Autodesk Fusion 360 part; units mm, degrees
(part 2 of 8)
  spline S26 degree 5 poles (-199.3182, -646.9433) (-199.2305, -646.913) (-199.0552, -646.8523) (-198.7925, -646.7608) (-198.4427, -646.6379) (-198.0064, -646.4828) (-197.571, -646.3262) (-197.1366, -646.1681) (-196.703, -646.0086) (-196.2703, -645.8476) (-195.8386, -645.6851) (-195.4078, -645.521) (-194.9779, -645.3555) (-194.549, -645.1885) (-194.1211, -645.0199) (-193.6942, -644.8498) (-193.2682, -644.6782) (-192.8433, -644.505) (-192.4194, -644.3303) (-191.9965, -644.154) (-191.5747, -643.9761) (-191.1539, -643.7966) (-190.7342, -643.6156) (-190.3155, -643.4329) (-189.898, -643.2486) (-189.4816, -643.0627) (-189.0663, -642.8752) (-188.6521, -642.686) (-188.2391, -642.4951) (-187.8273, -642.3026) (-187.4167, -642.1083) (-187.0073, -641.9124) (-186.599, -641.7148) (-186.1921, -641.5154) (-185.7864, -641.3143) (-185.382, -641.1114) (-184.9788, -640.9068) (-184.577, -640.7003) (-184.1766, -640.492) (-183.7775, -640.2819) (-183.3798, -640.07) (-182.9836, -639.8562) (-182.5887, -639.6404) (-182.1954, -639.4228) (-181.8035, -639.2033) (-181.4131, -638.9817) (-181.0244, -638.7582) (-180.6372, -638.5326) (-180.2517, -638.3049) (-179.8679, -638.0751) (-179.4858, -637.8433) (-179.1054, -637.6093) (-178.7267, -637.3731) (-178.3499, -637.1347) (-177.975, -636.8941) (-177.602, -636.651) (-177.2312, -636.4055) (-176.8625, -636.1574) (-176.4961, -635.9068) (-176.1319, -635.6535) (-175.77, -635.3976) (-175.4104, -635.1391) (-175.053, -634.8779) (-174.7334, -634.64) (-174.4864, -634.4531) (-174.3108, -634.3184) (-174.2058, -634.237) (-174.1705, -634.2097) knots -1 -1 -1 -1 -1 -1 -0.98571429 -0.97142857 -0.95714286 -0.94285714 -0.92857143 -0.91428571 -0.9 -0.88571429 -0.87142857 -0.85714286 -0.84285714 -0.82857143 -0.81428571 -0.8 -0.78571429 -0.77142857 -0.75714286 -0.74285714 -0.72857143 -0.71428571 -0.7 -0.68571429 -0.67142857 -0.65714286 -0.64285714 -0.62857143 -0.61428571 -0.6 -0.58571429 -0.57142857 -0.55714286 -0.54285714 -0.52857143 -0.51428571 -0.5 -0.48571429 -0.47142857 -0.45714286 -0.44285714 -0.42857143 -0.41428571 -0.4 -0.38571429 -0.37142857 -0.35714286 -0.34285714 -0.32857143 -0.31428571 -0.3 -0.28571429 -0.27142857 -0.25714286 -0.24285714 -0.22857143 -0.21428571 -0.2 -0.18571429 -0.17142857 -0.15714286 -0.14285714 -0.12857143 -0.11428571 -0.10707295 -0.10707295 -0.10707295 -0.10707295 -0.10707295 -0.10707295
  spline S27 degree 3 poles (-172.1165, -634.3004) (-172.268, -634.1598) (-172.4455, -634.05) (-172.8326, -633.9047) (-173.0384, -633.8705) (-173.412, -633.8819) (-173.5771, -633.9132) (-173.8914, -634.0263) (-174.0386, -634.1073) (-174.1705, -634.2097) knots 0 0 0 0 0.062015 0.062015 0.12403 0.12403 0.174133 0.174133 0.224236 0.224236 0.224236 0.224236
  arc A14 (-172.1165, -634.3004) -> (-165.887, -639.9095) centre (11.949, -436.1388) ccw
  spline S28 degree 3 poles (-165.5821, -641.9428) (-165.4731, -641.7671) (-165.3994, -641.5719) (-165.331, -641.1642) (-165.337, -640.9556) (-165.4198, -640.5911) (-165.4822, -640.4351) (-165.6535, -640.1483) (-165.7612, -640.0193) (-165.887, -639.9095) knots 0 0 0 0 0.062015 0.062015 0.12403 0.12403 0.174133 0.174133 0.224236 0.224236 0.224236 0.224236
  spline S29 degree 5 poles (-165.5821, -641.9428) (-165.6056, -641.9807) (-165.6755, -642.0937) (-165.7911, -642.2823) (-165.9512, -642.5475) (-166.1544, -642.8903) (-166.3768, -643.273) (-166.5963, -643.6576) (-166.8129, -644.0443) (-167.0268, -644.433) (-167.2378, -644.8236) (-167.4459, -645.2162) (-167.6513, -645.6106) (-167.8541, -646.0069) (-168.0542, -646.405) (-168.2519, -646.8047) (-168.4472, -647.2059) (-168.6402, -647.6087) (-168.8308, -648.013) (-169.0192, -648.4187) (-169.2053, -648.8259) (-169.3892, -649.2345) (-169.5709, -649.6445) (-169.7504, -650.0559) (-169.9278, -650.4685) (-170.1031, -650.8825) (-170.2764, -651.2977) (-170.4476, -651.7142) (-170.6169, -652.1319) (-170.7841, -652.5507) (-170.9494, -652.9707) (-171.1127, -653.3919) (-171.2741, -653.8142) (-171.4336, -654.2376) (-171.5912, -654.6621) (-171.7469, -655.0877) (-171.9008, -655.5143) (-172.0529, -655.942) (-172.2031, -656.3707) (-172.3515, -656.8004) (-172.4982, -657.2311) (-172.6431, -657.6627) (-172.7862, -658.0953) (-172.9275, -658.5289) (-173.0672, -658.9634) (-173.2051, -659.3989) (-173.3413, -659.8352) (-173.4758, -660.2724) (-173.6086, -660.7106) (-173.7397, -661.1495) (-173.8692, -661.5894) (-173.997, -662.0301) (-174.1232, -662.4716) (-174.2477, -662.914) (-174.3706, -663.3572) (-174.4919, -663.8012) (-174.6116, -664.246) (-174.7297, -664.6916) (-174.8462, -665.138) (-174.9611, -665.5851) (-175.0744, -666.033) (-175.1862, -666.4816) (-175.2964, -666.931) (-175.405, -667.3811) (-175.4907, -667.7418) (-175.5543, -668.0126) (-175.5964, -668.1933) (-175.6173, -668.2837) knots 0.10707295 0.10707295 0.10707295 0.10707295 0.10707295 0.10707295 0.11428571 0.12857143 0.14285714 0.15714286 0.17142857 0.18571429 0.2 0.21428571 0.22857143 0.24285714 0.25714286 0.27142857 0.28571429 0.3 0.31428571 0.32857143 0.34285714 0.35714286 0.37142857 0.38571429 0.4 0.41428571 0.42857143 0.44285714 0.45714286 0.47142857 0.48571429 0.5 0.51428571 0.52857143 0.54285714 0.55714286 0.57142857 0.58571429 0.6 0.61428571 0.62857143 0.64285714 0.65714286 0.67142857 0.68571429 0.7 0.71428571 0.72857143 0.74285714 0.75714286 0.77142857 0.78571429 0.8 0.81428571 0.82857143 0.84285714 0.85714286 0.87142857 0.88571429 0.9 0.91428571 0.92857143 0.94285714 0.95714286 0.97142857 0.98571429 1 1 1 1 1 1
  arc A15 (-175.6173, -668.2837) -> (-167.9238, -674.2945) centre (11.949, -436.1388) ccw
  spline S30 degree 5 poles (-167.9238, -674.2945) (-167.8412, -674.2523) (-167.6761, -674.1678) (-167.4286, -674.0406) (-167.0994, -673.8702) (-166.6889, -673.6559) (-166.2796, -673.4402) (-165.8713, -673.2232) (-165.4641, -673.0049) (-165.0581, -672.7852) (-164.6532, -672.5642) (-164.2494, -672.3418) (-163.8468, -672.1181) (-163.4453, -671.893) (-163.045, -671.6665) (-162.6459, -671.4387) (-162.248, -671.2094) (-161.8513, -670.9788) (-161.4558, -670.7468) (-161.0616, -670.5133) (-160.6686, -670.2785) (-160.2769, -670.0422) (-159.8865, -669.8045) (-159.4974, -669.5653) (-159.1095, -669.3247) (-158.723, -669.0827) (-158.3379, -668.8391) (-157.9541, -668.5941) (-157.5717, -668.3477) (-157.1907, -668.0997) (-156.811, -667.8502) (-156.4329, -667.5992) (-156.0561, -667.3467) (-155.6809, -667.0926) (-155.3071, -666.837) (-154.9349, -666.5798) (-154.5641, -666.321) (-154.195, -666.0607) (-153.8274, -665.7987) (-153.4615, -665.5351) (-153.0972, -665.2699) (-152.7345, -665.003) (-152.3735, -664.7344) (-152.0143, -664.4641) (-151.6568, -664.1922) (-151.3011, -663.9185) (-150.9472, -663.643) (-150.5952, -663.3657) (-150.2452, -663.0866) (-149.897, -662.8057) (-149.5509, -662.5229) (-149.2068, -662.2382) (-148.8647, -661.9516) (-148.5247, -661.6631) (-148.1869, -661.3726) (-147.8514, -661.0801) (-147.5183, -660.7853) (-147.1878, -660.4884) (-146.8598, -660.1891) (-146.5344, -659.8876) (-146.2117, -659.5838) (-145.8915, -659.2778) (-145.574, -658.9694) (-145.2905, -658.6894) (-145.072, -658.4699) (-144.9169, -658.3121) (-144.8242, -658.2169) (-144.7931, -658.1849) knots -1 -1 -1 -1 -1 -1 -0.98571429 -0.97142857 -0.95714286 -0.94285714 -0.92857143 -0.91428571 -0.9 -0.88571429 -0.87142857 -0.85714286 -0.84285714 -0.82857143 -0.81428571 -0.8 -0.78571429 -0.77142857 -0.75714286 -0.74285714 -0.72857143 -0.71428571 -0.7 -0.68571429 -0.67142857 -0.65714286 -0.64285714 -0.62857143 -0.61428571 -0.6 -0.58571429 -0.57142857 -0.55714286 -0.54285714 -0.52857143 -0.51428571 -0.5 -0.48571429 -0.47142857 -0.45714286 -0.44285714 -0.42857143 -0.41428571 -0.4 -0.38571429 -0.37142857 -0.35714286 -0.34285714 -0.32857143 -0.31428571 -0.3 -0.28571429 -0.27142857 -0.25714286 -0.24285714 -0.22857143 -0.21428571 -0.2 -0.18571429 -0.17142857 -0.15714286 -0.14285714 -0.12857143 -0.11428571 -0.10707295 -0.10707295 -0.10707295 -0.10707295 -0.10707295 -0.10707295
  spline S31 degree 3 poles (-142.7465, -657.9889) (-142.916, -657.8707) (-143.1071, -657.7867) (-143.5106, -657.6967) (-143.7192, -657.6915) (-144.0875, -657.7547) (-144.2467, -657.8088) (-144.5422, -657.9644) (-144.6767, -658.0651) (-144.7931, -658.1849) knots 0 0 0 0 0.062015 0.062015 0.12403 0.12403 0.174133 0.174133 0.224236 0.224236 0.224236 0.224236
  arc A16 (-142.7465, -657.9889) -> (-135.7969, -662.6764) centre (11.949, -436.1388) ccw
  spline S32 degree 3 poles (-135.212, -664.6475) (-135.1285, -664.4584) (-135.0827, -664.2548) (-135.0717, -663.8415) (-135.1067, -663.6357) (-135.2394, -663.2864) (-135.3229, -663.1406) (-135.5324, -662.8804) (-135.657, -662.7677) (-135.7969, -662.6764) knots 0 0 0 0 0.062015 0.062015 0.12403 0.12403 0.174133 0.174133 0.224236 0.224236 0.224236 0.224236
  spline S33 degree 5 poles (-135.212, -664.6475) (-135.23, -664.6882) (-135.2835, -664.8099) (-135.3717, -665.0128) (-135.4934, -665.2977) (-135.6468, -665.6654) (-135.8138, -666.0753) (-135.9776, -666.4868) (-136.1384, -666.8999) (-136.296, -667.3145) (-136.4506, -667.7306) (-136.6021, -668.1484) (-136.7506, -668.5676) (-136.8962, -668.9883) (-137.039, -669.4103) (-137.1792, -669.8336) (-137.3167, -670.2581) (-137.4518, -670.6839) (-137.5843, -671.1107) (-137.7144, -671.5387) (-137.842, -671.9679) (-137.9672, -672.3981) (-138.0901, -672.8294) (-138.2106, -673.2617) (-138.3289, -673.6951) (-138.4449, -674.1294) (-138.5587, -674.5647) (-138.6703, -675.0009) (-138.7797, -675.4381) (-138.887, -675.8761) (-138.9922, -676.3151) (-139.0954, -676.7549) (-139.1964, -677.1955) (-139.2954, -677.637) (-139.3924, -678.0793) (-139.4874, -678.5224) (-139.5804, -678.9663) (-139.6715, -679.411) (-139.7606, -679.8564) (-139.8478, -680.3026) (-139.9331, -680.7495) (-140.0164, -681.1971) (-140.0979, -681.6454) (-140.1776, -682.0945) (-140.2554, -682.5442) (-140.3314, -682.9946) (-140.4055, -683.4456) (-140.4778, -683.8973) (-140.5484, -684.3497) (-140.6172, -684.8026) (-140.6841, -685.2562) (-140.7494, -685.7104) (-140.8129, -686.1652) (-140.8746, -686.6206) (-140.9347, -687.0766) (-140.993, -687.5332) (-141.0496, -687.9903) (-141.1045, -688.448) (-141.1577, -688.9062) (-141.2093, -689.365) (-141.2592, -689.8243) (-141.3075, -690.2841) (-141.354, -690.7445) (-141.399, -691.2053) (-141.4337, -691.5744) (-141.4589, -691.8515) (-141.4754, -692.0363) (-141.4836, -692.1287) knots 0.10707295 0.10707295 0.10707295 0.10707295 0.10707295 0.10707295 0.11428571 0.12857143 0.14285714 0.15714286 0.17142857 0.18571429 0.2 0.21428571 0.22857143 0.24285714 0.25714286 0.27142857 0.28571429 0.3 0.31428571 0.32857143 0.34285714 0.35714286 0.37142857 0.38571429 0.4 0.41428571 0.42857143 0.44285714 0.45714286 0.47142857 0.48571429 0.5 0.51428571 0.52857143 0.54285714 0.55714286 0.57142857 0.58571429 0.6 0.61428571 0.62857143 0.64285714 0.65714286 0.67142857 0.68571429 0.7 0.71428571 0.72857143 0.74285714 0.75714286 0.77142857 0.78571429 0.8 0.81428571 0.82857143 0.84285714 0.85714286 0.87142857 0.88571429 0.9 0.91428571 0.92857143 0.94285714 0.95714286 0.97142857 0.98571429 1 1 1 1 1 1
  arc A17 (-141.4836, -692.1287) -> (-133.0285, -697.0103) centre (11.949, -436.1388) ccw
  spline S34 degree 5 poles (-133.0285, -697.0103) (-132.9525, -696.957) (-132.8007, -696.8503) (-132.5734, -696.6899) (-132.2711, -696.4753) (-131.8945, -696.2059) (-131.5191, -695.9354) (-131.145, -695.6637) (-130.7722, -695.3909) (-130.4007, -695.1168) (-130.0304, -694.8416) (-129.6615, -694.5652) (-129.2939, -694.2876) (-128.9277, -694.0088) (-128.5628, -693.7289) (-128.1993, -693.4477) (-127.8372, -693.1653) (-127.4765, -692.8817) (-127.1171, -692.5969) (-126.7592, -692.3108) (-126.4028, -692.0236) (-126.0478, -691.7351) (-125.6942, -691.4453) (-125.3422, -691.1543) (-124.9916, -690.8621) (-124.6425, -690.5686) (-124.295, -690.2739) (-123.9491, -689.9778) (-123.6047, -689.6805) (-123.2619, -689.3819) (-122.9207, -689.0821) (-122.5811, -688.7809) (-122.2432, -688.4784) (-121.907, -688.1746) (-121.5724, -687.8694) (-121.2396, -687.5629) (-120.9085, -687.2551) (-120.5791, -686.9459) (-120.2516, -686.6353) (-119.9259, -686.3233) (-119.6021, -686.01) (-119.2801, -685.6952) (-118.96, -685.379) (-118.6418, -685.0614) (-118.3257, -684.7423) (-118.0115, -684.4218) (-117.6994, -684.0997) (-117.3895, -683.7761) (-117.0817, -683.451) (-116.776, -683.1244) (-116.4726, -682.7962) (-116.1715, -682.4664) (-115.8726, -682.135) (-115.576, -681.802) (-115.282, -681.4673) (-114.9905, -681.1309) (-114.7016, -680.7926) (-114.4156, -680.4526) (-114.1325, -680.1106) (-113.8523, -679.7667) (-113.5749, -679.421) (-113.3005, -679.0734) (-113.029, -678.7238) (-112.7872, -678.4071) (-112.6013, -678.1593) (-112.4697, -677.9814) (-112.3912, -677.8742) (-112.3648, -677.8383) knots -1 -1 -1 -1 -1 -1 -0.98571429 -0.97142857 -0.95714286 -0.94285714 -0.92857143 -0.91428571 -0.9 -0.88571429 -0.87142857 -0.85714286 -0.84285714 -0.82857143 -0.81428571 -0.8 -0.78571429 -0.77142857 -0.75714286 -0.74285714 -0.72857143 -0.71428571 -0.7 -0.68571429 -0.67142857 -0.65714286 -0.64285714 -0.62857143 -0.61428571 -0.6 -0.58571429 -0.57142857 -0.55714286 -0.54285714 -0.52857143 -0.51428571 -0.5 -0.48571429 -0.47142857 -0.45714286 -0.44285714 -0.42857143 -0.41428571 -0.4 -0.38571429 -0.37142857 -0.35714286 -0.34285714 -0.32857143 -0.31428571 -0.3 -0.28571429 -0.27142857 -0.25714286 -0.24285714 -0.22857143 -0.21428571 -0.2 -0.18571429 -0.17142857 -0.15714286 -0.14285714 -0.12857143 -0.11428571 -0.10707295 -0.10707295 -0.10707295 -0.10707295 -0.10707295 -0.10707295
  spline S35 degree 3 poles (-110.3654, -677.3593) (-110.5498, -677.2658) (-110.7506, -677.2093) (-111.1627, -677.1763) (-111.3701, -677.2002) (-111.726, -677.314) (-111.8761, -677.3897) (-112.147, -677.585) (-112.2663, -677.7034) (-112.3648, -677.8383) knots 0 0 0 0 0.062015 0.062015 0.12403 0.12403 0.174133 0.174133 0.224236 0.224236 0.224236 0.224236
  arc A18 (-110.3654, -677.3593) -> (-102.8311, -681.034) centre (11.949, -436.1388) ccw
  spline S36 degree 3 poles (-101.9775, -682.9045) (-101.9212, -682.7056) (-101.9042, -682.4976) (-101.9508, -682.0868) (-102.0141, -681.888) (-102.1941, -681.5604) (-102.2972, -681.4277) (-102.5408, -681.1992) (-102.6799, -681.1049) (-102.8311, -681.034) knots 0 0 0 0 0.062015 0.062015 0.12403 0.12403 0.174133 0.174133 0.224236 0.224236 0.224236 0.224236
  spline S37 degree 5 poles (-101.9775, -682.9045) (-101.9897, -682.9474) (-102.0258, -683.0753) (-102.0849, -683.2885) (-102.1657, -683.5875) (-102.2665, -683.973) (-102.3748, -684.4022) (-102.4798, -684.8325) (-102.5815, -685.2639) (-102.6799, -685.6964) (-102.7751, -686.1301) (-102.8669, -686.5648) (-102.9557, -687.0006) (-103.0413, -687.4375) (-103.124, -687.8752) (-103.2038, -688.3139) (-103.281, -688.7535) (-103.3554, -689.1938) (-103.4273, -689.635) (-103.4965, -690.077) (-103.5632, -690.5197) (-103.6273, -690.9631) (-103.689, -691.4073) (-103.7482, -691.8522) (-103.8049, -692.2978) (-103.8594, -692.7441) (-103.9115, -693.191) (-103.9613, -693.6385) (-104.0088, -694.0866) (-104.0541, -694.5353) (-104.0972, -694.9846) (-104.1381, -695.4345) (-104.1769, -695.885) (-104.2135, -696.3359) (-104.248, -696.7874) (-104.2803, -697.2394) (-104.3107, -697.692) (-104.339, -698.145) (-104.3652, -698.5985) (-104.3895, -699.0524) (-104.4117, -699.5069) (-104.432, -699.9617) (-104.4503, -700.417) (-104.4667, -700.8728) (-104.4811, -701.3289) (-104.4937, -701.7855) (-104.5043, -702.2425) (-104.5131, -702.6999) (-104.52, -703.1576) (-104.5251, -703.6158) (-104.5283, -704.0743) (-104.5297, -704.5331) (-104.5293, -704.9923) (-104.527, -705.4519) (-104.523, -705.9118) (-104.5172, -706.372) (-104.5097, -706.8326) (-104.5003, -707.2935) (-104.4893, -707.7546) (-104.4765, -708.2161) (-104.462, -708.6779) (-104.4458, -709.14) (-104.4278, -709.6023) (-104.4082, -710.0649) (-104.3912, -710.4353) (-104.3776, -710.7131) (-104.3683, -710.8984) (-104.3635, -710.9911) knots 0.10707295 0.10707295 0.10707295 0.10707295 0.10707295 0.10707295 0.11428571 0.12857143 0.14285714 0.15714286 0.17142857 0.18571429 0.2 0.21428571 0.22857143 0.24285714 0.25714286 0.27142857 0.28571429 0.3 0.31428571 0.32857143 0.34285714 0.35714286 0.37142857 0.38571429 0.4 0.41428571 0.42857143 0.44285714 0.45714286 0.47142857 0.48571429 0.5 0.51428571 0.52857143 0.54285714 0.55714286 0.57142857 0.58571429 0.6 0.61428571 0.62857143 0.64285714 0.65714286 0.67142857 0.68571429 0.7 0.71428571 0.72857143 0.74285714 0.75714286 0.77142857 0.78571429 0.8 0.81428571 0.82857143 0.84285714 0.85714286 0.87142857 0.88571429 0.9 0.91428571 0.92857143 0.94285714 0.95714286 0.97142857 0.98571429 1 1 1 1 1 1
  arc A19 (-104.3635, -710.9911) -> (-95.3113, -714.6484) centre (11.949, -436.1388) ccw
  spline S38 degree 5 poles (-95.3113, -714.6484) (-95.2435, -714.5851) (-95.108, -714.4583) (-94.9052, -714.2678) (-94.6357, -714.0133) (-94.3002, -713.6941) (-93.9662, -713.374) (-93.6335, -713.0529) (-93.3023, -712.7308) (-92.9725, -712.4077) (-92.6442, -712.0836) (-92.3174, -711.7586) (-91.992, -711.4325) (-91.6681, -711.1055) (-91.3458, -710.7775) (-91.0249, -710.4484) (-90.7056, -710.1184) (-90.3879, -709.7874) (-90.0717, -709.4553) (-89.7571, -709.1222) (-89.4441, -708.7882) (-89.1327, -708.4531) (-88.8229, -708.1169) (-88.5147, -707.7798) (-88.2083, -707.4416) (-87.9034, -707.1024) (-87.6003, -706.7622) (-87.2989, -706.4209) (-86.9993, -706.0785) (-86.7014, -705.7351) (-86.4052, -705.3907) (-86.1109, -705.0452) (-85.8184, -704.6986) (-85.5277, -704.3509) (-85.2388, -704.0022) (-84.9519, -703.6523) (-84.6669, -703.3014) (-84.3838, -702.9494) (-84.1027, -702.5962) (-83.8236, -702.242) (-83.5465, -701.8866) (-83.2714, -701.5301) (-82.9985, -701.1724) (-82.7276, -700.8136) (-82.4589, -700.4536) (-82.1924, -700.0925) (-81.9282, -699.7301) (-81.6663, -699.3666) (-81.4067, -699.0018) (-81.1495, -698.6358) (-80.8948, -698.2685) (-80.6424, -697.9001) (-80.3926, -697.5303) (-80.1453, -697.1592) (-79.9006, -696.7869) (-79.6588, -696.4132) (-79.4198, -696.038) (-79.184, -695.6615) (-78.9512, -695.2834) (-78.7215, -694.9039) (-78.495, -694.523) (-78.2716, -694.1405) (-78.0514, -693.7566) (-77.8561, -693.4093) (-77.7065, -693.138) (-77.6009, -692.9435) (-77.538, -692.8265) (-77.517, -692.7872) knots -1 -1 -1 -1 -1 -1 -0.98571429 -0.97142857 -0.95714286 -0.94285714 -0.92857143 -0.91428571 -0.9 -0.88571429 -0.87142857 -0.85714286 -0.84285714 -0.82857143 -0.81428571 -0.8 -0.78571429 -0.77142857 -0.75714286 -0.74285714 -0.72857143 -0.71428571 -0.7 -0.68571429 -0.67142857 -0.65714286 -0.64285714 -0.62857143 -0.61428571 -0.6 -0.58571429 -0.57142857 -0.55714286 -0.54285714 -0.52857143 -0.51428571 -0.5 -0.48571429 -0.47142857 -0.45714286 -0.44285714 -0.42857143 -0.41428571 -0.4 -0.38571429 -0.37142857 -0.35714286 -0.34285714 -0.32857143 -0.31428571 -0.3 -0.28571429 -0.27142857 -0.25714286 -0.24285714 -0.22857143 -0.21428571 -0.2 -0.18571429 -0.17142857 -0.15714286 -0.14285714 -0.12857143 -0.11428571 -0.10707295 -0.10707295 -0.10707295 -0.10707295 -0.10707295 -0.10707295
  spline S39 degree 3 poles (-75.6036, -692.0347) (-75.7992, -691.9678) (-76.006, -691.9397) (-76.4187, -691.9644) (-76.6207, -692.0169) (-76.9573, -692.1792) (-77.0954, -692.275) (-77.3365, -692.5061) (-77.4381, -692.64) (-77.517, -692.7872) knots 0 0 0 0 0.062015 0.062015 0.12403 0.12403 0.174133 0.174133 0.224236 0.224236 0.224236 0.224236
  arc A20 (-75.6036, -692.0347) -> (-67.6313, -694.625) centre (11.949, -436.1388) ccw
  spline S40 degree 3 poles (-66.5257, -696.3585) (-66.4975, -696.1537) (-66.5096, -695.9454) (-66.613, -695.5451) (-66.7033, -695.3569) (-66.9272, -695.0577) (-67.0477, -694.9406) (-67.3208, -694.7482) (-67.4716, -694.6742) (-67.6313, -694.625) knots 0 0 0 0 0.062015 0.062015 0.12403 0.12403 0.174133 0.174133 0.224236 0.224236 0.224236 0.224236
  spline S41 degree 5 poles (-66.5257, -696.3585) (-66.5317, -696.4026) (-66.5496, -696.5343) (-66.5785, -696.7537) (-66.617, -697.0611) (-66.6631, -697.4569) (-66.7106, -697.8969) (-66.7547, -698.3376) (-66.7953, -698.779) (-66.8326, -699.221) (-66.8665, -699.6637) (-66.897, -700.107) (-66.9242, -700.5509) (-66.9482, -700.9954) (-66.9692, -701.4404) (-66.9872, -701.886) (-67.0024, -702.332) (-67.0148, -702.7784) (-67.0246, -703.2253) (-67.0316, -703.6726) (-67.0361, -704.1202) (-67.0379, -704.5683) (-67.0371, -705.0168) (-67.0338, -705.4656) (-67.028, -705.9147) (-67.0198, -706.3642) (-67.0092, -706.814) (-66.9962, -707.2641) (-66.9809, -707.7145) (-66.9633, -708.1652) (-66.9435, -708.6161) (-66.9214, -709.0673) (-66.897, -709.5187) (-66.8705, -709.9704) (-66.8418, -710.4223) (-66.811, -710.8744) (-66.7781, -711.3268) (-66.743, -711.7793) (-66.7059, -712.232) (-66.6668, -712.685) (-66.6255, -713.1381) (-66.5823, -713.5913) (-66.5371, -714.0448) (-66.4899, -714.4983) (-66.4407, -714.9521) (-66.3896, -715.406) (-66.3365, -715.86) (-66.2816, -716.3141) (-66.2247, -716.7684) (-66.1659, -717.2227) (-66.1053, -717.6772) (-66.0428, -718.1318) (-65.9785, -718.5865) (-65.9123, -719.0413) (-65.8444, -719.4962) (-65.7746, -719.9511) (-65.703, -720.4061) (-65.6296, -720.8612) (-65.5545, -721.3164) (-65.4776, -721.7716) (-65.399, -722.2268) (-65.3186, -722.6822) (-65.2365, -723.1375) (-65.1527, -723.5929) (-65.0843, -723.9573) (-65.0322, -724.2305) (-64.9971, -724.4127) (-64.9795, -724.5038) knots 0.10707295 0.10707295 0.10707295 0.10707295 0.10707295 0.10707295 0.11428571 0.12857143 0.14285714 0.15714286 0.17142857 0.18571429 0.2 0.21428571 0.22857143 0.24285714 0.25714286 0.27142857 0.28571429 0.3 0.31428571 0.32857143 0.34285714 0.35714286 0.37142857 0.38571429 0.4 0.41428571 0.42857143 0.44285714 0.45714286 0.47142857 0.48571429 0.5 0.51428571 0.52857143 0.54285714 0.55714286 0.57142857 0.58571429 0.6 0.61428571 0.62857143 0.64285714 0.65714286 0.67142857 0.68571429 0.7 0.71428571 0.72857143 0.74285714 0.75714286 0.77142857 0.78571429 0.8 0.81428571 0.82857143 0.84285714 0.85714286 0.87142857 0.88571429 0.9 0.91428571 0.92857143 0.94285714 0.95714286 0.97142857 0.98571429 1 1 1 1 1 1
  arc A21 (-64.9795, -724.5038) -> (-55.5064, -726.8657) centre (11.949, -436.1388) ccw
  spline S42 degree 5 poles (-55.5064, -726.8657) (-55.448, -726.7936) (-55.3315, -726.6492) (-55.1572, -726.4323) (-54.9258, -726.1428) (-54.638, -725.78) (-54.3517, -725.4165) (-54.067, -725.0522) (-53.7838, -724.6872) (-53.5022, -724.3213) (-53.2222, -723.9547) (-52.9438, -723.5874) (-52.667, -723.2192) (-52.3918, -722.8503) (-52.1182, -722.4806) (-51.8463, -722.1101) (-51.576, -721.7388) (-51.3074, -721.3668) (-51.0405, -720.9939) (-50.7753, -720.6203) (-50.5119, -720.2459) (-50.2501, -719.8708) (-49.9901, -719.4948) (-49.7319, -719.118) (-49.4755, -718.7405) (-49.2208, -718.3622) (-48.968, -717.9831) (-48.7171, -717.6031) (-48.468, -717.2224) (-48.2208, -716.8409) (-47.9754, -716.4586) (-47.732, -716.0755) (-47.4906, -715.6915) (-47.2511, -715.3068) (-47.0136, -714.9213) (-46.7782, -714.5349) (-46.5448, -714.1477) (-46.3134, -713.7597) (-46.0842, -713.3709) (-45.8571, -712.9813) (-45.6322, -712.5908) (-45.4094, -712.1994) (-45.1889, -711.8073) (-44.9706, -711.4143) (-44.7546, -711.0204) (-44.541, -710.6257) (-44.3298, -710.2301) (-44.121, -709.8336) (-43.9147, -709.4363) (-43.711, -709.038) (-43.5098, -708.6389) (-43.3112, -708.2388) (-43.1152, -707.8379) (-42.922, -707.4361) (-42.7315, -707.0333) (-42.5441, -706.6295) (-42.3597, -706.2248) (-42.1785, -705.8191) (-42.0006, -705.4123) (-41.826, -705.0045) (-41.6547, -704.5957) (-41.4866, -704.1859) (-41.322, -703.7751) (-41.177, -703.404) (-41.0666, -703.1145) (-40.9891, -702.9073) (-40.9431, -702.7826) (-40.9277, -702.7408) knots -1 -1 -1 -1 -1 -1 -0.98571429 -0.97142857 -0.95714286 -0.94285714 -0.92857143 -0.91428571 -0.9 -0.88571429 -0.87142857 -0.85714286 -0.84285714 -0.82857143 -0.81428571 -0.8 -0.78571429 -0.77142857 -0.75714286 -0.74285714 -0.72857143 -0.71428571 -0.7 -0.68571429 -0.67142857 -0.65714286 -0.64285714 -0.62857143 -0.61428571 -0.6 -0.58571429 -0.57142857 -0.55714286 -0.54285714 -0.52857143 -0.51428571 -0.5 -0.48571429 -0.47142857 -0.45714286 -0.44285714 -0.42857143 -0.41428571 -0.4 -0.38571429 -0.37142857 -0.35714286 -0.34285714 -0.32857143 -0.31428571 -0.3 -0.28571429 -0.27142857 -0.25714286 -0.24285714 -0.22857143 -0.21428571 -0.2 -0.18571429 -0.17142857 -0.15714286 -0.14285714 -0.12857143 -0.11428571 -0.10707295 -0.10707295 -0.10707295 -0.10707295 -0.10707295 -0.10707295
  spline S43 degree 3 poles (-39.1377, -701.7293) (-39.3407, -701.6902) (-39.5494, -701.6912) (-39.9547, -701.7731) (-40.1473, -701.8532) (-40.4581, -702.0608) (-40.5815, -702.1749) (-40.7882, -702.4373) (-40.8701, -702.584) (-40.9277, -702.7408) knots 0 0 0 0 0.062015 0.062015 0.12403 0.12403 0.174133 0.174133 0.224236 0.224236 0.224236 0.224236
  arc A22 (-39.1377, -701.7293) -> (-30.8825, -703.1849) centre (11.949, -436.1388) ccw
  spline S44 degree 3 poles (-29.5464, -704.7476) (-29.547, -704.5409) (-29.588, -704.3363) (-29.7461, -703.9543) (-29.8617, -703.7805) (-30.125, -703.5153) (-30.2607, -703.4161) (-30.5579, -703.2637) (-30.7176, -703.2114) (-30.8825, -703.1849) knots 0 0 0 0 0.062015 0.062015 0.12403 0.12403 0.174133 0.174133 0.224236 0.224236 0.224236 0.224236
  spline S45 degree 5 poles (-29.5464, -704.7476) (-29.5462, -704.7922) (-29.5456, -704.9251) (-29.5437, -705.1463) (-29.539, -705.4561) (-29.5296, -705.8544) (-29.5154, -706.2968) (-29.4977, -706.7393) (-29.4766, -707.1821) (-29.452, -707.625) (-29.4239, -708.068) (-29.3924, -708.5113) (-29.3576, -708.9547) (-29.3195, -709.3982) (-29.2783, -709.8418) (-29.2341, -710.2855) (-29.1871, -710.7293) (-29.1373, -711.1731) (-29.0847, -711.617) (-29.0295, -712.0609) (-28.9716, -712.5049) (-28.911, -712.9488) (-28.8478, -713.3928) (-28.7821, -713.8368) (-28.7138, -714.2808) (-28.6431, -714.7247) (-28.57, -715.1687) (-28.4945, -715.6126) (-28.4167, -716.0565) (-28.3366, -716.5003) (-28.2542, -716.9441) (-28.1695, -717.3878) (-28.0826, -717.8314) (-27.9935, -718.275) (-27.9022, -718.7186) (-27.8087, -719.162) (-27.7131, -719.6053) (-27.6155, -720.0486) (-27.5157, -720.4918) (-27.4139, -720.9348) (-27.31, -721.3778) (-27.2041, -721.8206) (-27.0962, -722.2633) (-26.9864, -722.7059) (-26.8745, -723.1484) (-26.7607, -723.5908) (-26.645, -724.033) (-26.5274, -724.4751) (-26.4078, -724.917) (-26.2864, -725.3588) (-26.1631, -725.8004) (-26.038, -726.2419) (-25.911, -726.6832) (-25.7822, -727.1243) (-25.6516, -727.5653) (-25.5191, -728.0061) (-25.3849, -728.4467) (-25.2489, -728.8872) (-25.1112, -729.3274) (-24.9717, -729.7675) (-24.8305, -730.2074) (-24.6875, -730.6471) (-24.5428, -731.0866) (-24.3965, -731.5259) (-24.278, -731.8772) (-24.1884, -732.1406) (-24.1283, -732.3161) (-24.0982, -732.4039) knots 0.10707295 0.10707295 0.10707295 0.10707295 0.10707295 0.10707295 0.11428571 0.12857143 0.14285714 0.15714286 0.17142857 0.18571429 0.2 0.21428571 0.22857143 0.24285714 0.25714286 0.27142857 0.28571429 0.3 0.31428571 0.32857143 0.34285714 0.35714286 0.37142857 0.38571429 0.4 0.41428571 0.42857143 0.44285714 0.45714286 0.47142857 0.48571429 0.5 0.51428571 0.52857143 0.54285714 0.55714286 0.57142857 0.58571429 0.6 0.61428571 0.62857143 0.64285714 0.65714286 0.67142857 0.68571429 0.7 0.71428571 0.72857143 0.74285714 0.75714286 0.77142857 0.78571429 0.8 0.81428571 0.82857143 0.84285714 0.85714286 0.87142857 0.88571429 0.9 0.91428571 0.92857143 0.94285714 0.95714286 0.97142857 0.98571429 1 1 1 1 1 1
  arc A23 (-24.0982, -732.4039) -> (-14.3885, -733.4244) centre (11.949, -436.1388) ccw
  spline S46 degree 5 poles (-14.3885, -733.4244) (-14.3408, -733.3448) (-14.2455, -733.1856) (-14.1031, -732.9466) (-13.9142, -732.6276) (-13.6797, -732.2284) (-13.4468, -731.8286) (-13.2156, -731.4282) (-12.986, -731.0273) (-12.758, -730.6258) (-12.5317, -730.2238) (-12.3071, -729.8213) (-12.0843, -729.4182) (-11.8631, -729.0145) (-11.6436, -728.6103) (-11.4259, -728.2056) (-11.2099, -727.8003) (-10.9957, -727.3945) (-10.7833, -726.9882) (-10.5727, -726.5813) (-10.3639, -726.1739) (-10.1569, -725.7659) (-9.9518, -725.3575) (-9.7485, -724.9484) (-9.5471, -724.5389) (-9.3476, -724.1288) (-9.15, -723.7182) (-8.9544, -723.307) (-8.7607, -722.8954) (-8.569, -722.4831) (-8.3793, -722.0704) (-8.1916, -721.6571) (-8.0059, -721.2434) (-7.8223, -720.829) (-7.6408, -720.4142) (-7.4614, -719.9988) (-7.2841, -719.5829) (-7.109, -719.1665) (-6.9362, -718.7496) (-6.7655, -718.3321) (-6.5971, -717.9141) (-6.431, -717.4956) (-6.2672, -717.0765) (-6.1057, -716.657) (-5.9467, -716.2369) (-5.7901, -715.8163) (-5.6359, -715.3951) (-5.4844, -714.9735) (-5.3354, -714.5513) (-5.1891, -714.1285) (-5.0454, -713.7053) (-4.9044, -713.2815) (-4.7661, -712.8572) (-4.6307, -712.4324) (-4.4982, -712.007) (-4.3687, -711.5811) (-4.2424, -711.1547) (-4.1195, -710.7277) (-3.9999, -710.3001) (-3.8838, -709.872) (-3.771, -709.4433) (-3.6617, -709.0141) (-3.5558, -708.5844) (-3.4638, -708.1967) (-3.3948, -707.8947) (-3.3469, -707.6787) (-3.3187, -707.5488) (-3.3093, -707.5052) knots -1 -1 -1 -1 -1 -1 -0.98571429 -0.97142857 -0.95714286 -0.94285714 -0.92857143 -0.91428571 -0.9 -0.88571429 -0.87142857 -0.85714286 -0.84285714 -0.82857143 -0.81428571 -0.8 -0.78571429 -0.77142857 -0.75714286 -0.74285714 -0.72857143 -0.71428571 -0.7 -0.68571429 -0.67142857 -0.65714286 -0.64285714 -0.62857143 -0.61428571 -0.6 -0.58571429 -0.57142857 -0.55714286 -0.54285714 -0.52857143 -0.51428571 -0.5 -0.48571429 -0.47142857 -0.45714286 -0.44285714 -0.42857143 -0.41428571 -0.4 -0.38571429 -0.37142857 -0.35714286 -0.34285714 -0.32857143 -0.31428571 -0.3 -0.28571429 -0.27142857 -0.25714286 -0.24285714 -0.22857143 -0.21428571 -0.2 -0.18571429 -0.17142857 -0.15714286 -0.14285714 -0.12857143 -0.11428571 -0.10707295 -0.10707295 -0.10707295 -0.10707295 -0.10707295 -0.10707295
  spline S47 degree 3 poles (-1.6775, -706.2545) (-1.884, -706.2441) (-2.0905, -706.2741) (-2.4804, -706.4116) (-2.66, -706.5177) (-2.9389, -706.7665) (-3.0452, -706.8967) (-3.2133, -707.1853) (-3.2741, -707.342) (-3.3093, -707.5052) knots 0 0 0 0 0.062015 0.062015 0.12403 0.12403 0.174133 0.174133 0.224236 0.224236 0.224236 0.224236
  arc A24 (-1.6775, -706.2545) -> (6.7, -706.547) centre (11.949, -436.1388) ccw
  spline S48 degree 3 poles (8.2406, -707.9086) (8.2112, -707.7039) (8.1421, -707.507) (7.9324, -707.1507) (7.7937, -706.9948) (7.4961, -706.7688) (7.3479, -706.6895) (7.0324, -706.5798) (6.867, -706.5503) (6.7, -706.547) knots 0 0 0 0 0.062015 0.062015 0.12403 0.12403 0.174133 0.174133 0.224236 0.224236 0.224236 0.224236
  spline S49 degree 5 poles (8.2406, -707.9086) (8.2469, -707.9527) (8.266, -708.0842) (8.2987, -708.303) (8.3465, -708.6091) (8.4112, -709.0023) (8.4868, -709.4384) (8.566, -709.8741) (8.6485, -710.3096) (8.7345, -710.7448) (8.824, -711.1796) (8.9169, -711.6142) (9.0131, -712.0484) (9.1125, -712.4823) (9.2151, -712.9159) (9.3205, -713.3491) (9.4289, -713.782) (9.5399, -714.2146) (9.6537, -714.6469) (9.7702, -715.0788) (9.8894, -715.5103) (10.0112, -715.9415) (10.1355, -716.3724) (10.2624, -716.8029) (10.3918, -717.2331) (10.5236, -717.6629) (10.6578, -718.0923) (10.7943, -718.5214) (10.9331, -718.9501) (11.0742, -719.3785) (11.2176, -719.8065) (11.3632, -720.2341) (11.511, -720.6614) (11.661, -721.0882) (11.8132, -721.5147) (11.9674, -721.9408) (12.1238, -722.3666) (12.2822, -722.7919) (12.4427, -723.2169) (12.6052, -723.6415) (12.7697, -724.0657) (12.9361, -724.4894) (13.1046, -724.9128) (13.275, -725.3358) (13.4473, -725.7585) (13.6216, -726.1807) (13.7977, -726.6025) (13.9757, -727.0239) (14.1556, -727.4448) (14.3373, -727.8654) (14.5209, -728.2856) (14.7063, -728.7054) (14.8934, -729.1247) (15.0824, -729.5436) (15.2731, -729.9621) (15.4656, -730.3802) (15.6598, -730.7979) (15.8558, -731.2151) (16.0535, -731.6319) (16.2528, -732.0483) (16.4539, -732.4643) (16.6567, -732.8798) (16.8611, -733.2949) (17.0672, -733.7095) (17.2334, -734.0409) (17.3588, -734.2892) (17.4427, -734.4547) (17.4848, -734.5374) knots 0.10707295 0.10707295 0.10707295 0.10707295 0.10707295 0.10707295 0.11428571 0.12857143 0.14285714 0.15714286 0.17142857 0.18571429 0.2 0.21428571 0.22857143 0.24285714 0.25714286 0.27142857 0.28571429 0.3 0.31428571 0.32857143 0.34285714 0.35714286 0.37142857 0.38571429 0.4 0.41428571 0.42857143 0.44285714 0.45714286 0.47142857 0.48571429 0.5 0.51428571 0.52857143 0.54285714 0.55714286 0.57142857 0.58571429 0.6 0.61428571 0.62857143 0.64285714 0.65714286 0.67142857 0.68571429 0.7 0.71428571 0.72857143 0.74285714 0.75714286 0.77142857 0.78571429 0.8 0.81428571 0.82857143 0.84285714 0.85714286 0.87142857 0.88571429 0.9 0.91428571 0.92857143 0.94285714 0.95714286 0.97142857 0.98571429 1 1 1 1 1 1
  arc A25 (17.4848, -734.5374) -> (27.242, -734.1967) centre (11.949, -436.1388) ccw
  spline S50 degree 5 poles (27.242, -734.1967) (27.2781, -734.1112) (27.3503, -733.9403) (27.4581, -733.6838) (27.6008, -733.3417) (27.7774, -732.9137) (27.9524, -732.4853) (28.1257, -732.0567) (28.2973, -731.6277) (28.4671, -731.1984) (28.6352, -730.7689) (28.8016, -730.339) (28.9662, -729.9088) (29.1291, -729.4783) (29.2902, -729.0475) (29.4494, -728.6164) (29.6069, -728.185) (29.7625, -727.7533) (29.9163, -727.3214) (30.0683, -726.8892) (30.2183, -726.4567) (30.3665, -726.0239) (30.5128, -725.5908) (30.6572, -725.1575) (30.7996, -724.7239) (30.9401, -724.29) (31.0786, -723.8559) (31.2151, -723.4215) (31.3496, -722.9869) (31.4821, -722.552) (31.6125, -722.1169) (31.7409, -721.6815) (31.8672, -721.2459) (31.9913, -720.8101) (32.1134, -720.374) (32.2332, -719.9377) (32.3508, -719.5012) (32.4663, -719.0645) (32.5794, -718.6275) (32.6903, -718.1904) (32.7989, -717.753) (32.9052, -717.3154) (33.0091, -716.8777) (33.1106, -716.4397) (33.2096, -716.0016) (33.3062, -715.5633) (33.4002, -715.1248) (33.4916, -714.6861) (33.5803, -714.2473) (33.6664, -713.8083) (33.7498, -713.3692) (33.8304, -712.9299) (33.9083, -712.4905) (33.9833, -712.051) (34.0553, -711.6113) (34.1243, -711.1715) (34.19, -710.7316) (34.2523, -710.2917) (34.3112, -709.8516) (34.3666, -709.4115) (34.4186, -708.9714) (34.4672, -708.5311) (34.5122, -708.0908) (34.5493, -707.6941) (34.5756, -707.3854) (34.593, -707.1648) (34.6029, -707.0323) (34.6061, -706.9879) knots -1 -1 -1 -1 -1 -1 -0.98571429 -0.97142857 -0.95714286 -0.94285714 -0.92857143 -0.91428571 -0.9 -0.88571429 -0.87142857 -0.85714286 -0.84285714 -0.82857143 -0.81428571 -0.8 -0.78571429 -0.77142857 -0.75714286 -0.74285714 -0.72857143 -0.71428571 -0.7 -0.68571429 -0.67142857 -0.65714286 -0.64285714 -0.62857143 -0.61428571 -0.6 -0.58571429 -0.57142857 -0.55714286 -0.54285714 -0.52857143 -0.51428571 -0.5 -0.48571429 -0.47142857 -0.45714286 -0.44285714 -0.42857143 -0.41428571 -0.4 -0.38571429 -0.37142857 -0.35714286 -0.34285714 -0.32857143 -0.31428571 -0.3 -0.28571429 -0.27142857 -0.25714286 -0.24285714 -0.22857143 -0.21428571 -0.2 -0.18571429 -0.17142857 -0.15714286 -0.14285714 -0.12857143 -0.11428571 -0.10707295 -0.10707295 -0.10707295 -0.10707295 -0.10707295 -0.10707295
  spline S51 degree 3 poles (36.0479, -705.5222) (35.842, -705.5406) (35.6417, -705.599) (35.2747, -705.7895) (35.1116, -705.9196) (34.8701, -706.2048) (34.7829, -706.3485) (34.6566, -706.6577) (34.6182, -706.8213) (34.6061, -706.9879) knots 0 0 0 0 0.062015 0.062015 0.12403 0.12403 0.174133 0.174133 0.224236 0.224236 0.224236 0.224236
  arc A26 (36.0479, -705.5222) -> (44.3847, -704.6459) centre (11.949, -436.1388) ccw
  spline S52 degree 3 poles (46.0997, -705.7798) (46.0421, -705.5813) (45.9463, -705.3959) (45.6891, -705.0723) (45.5301, -704.9371) (45.2038, -704.7548) (45.0461, -704.6968) (44.7184, -704.6322) (44.5505, -704.6259) (44.3847, -704.6459) knots 0 0 0 0 0.062015 0.062015 0.12403 0.12403 0.174133 0.174133 0.224236 0.224236 0.224236 0.224236
  spline S53 degree 5 poles (46.0997, -705.7798) (46.1121, -705.8226) (46.1493, -705.9502) (46.2122, -706.1624) (46.3021, -706.4588) (46.4209, -706.8392) (46.5565, -707.2605) (46.6955, -707.681) (46.8379, -708.1007) (46.9836, -708.5197) (47.1327, -708.9379) (47.2851, -709.3553) (47.4409, -709.7719) (47.5997, -710.1877) (47.7616, -710.6028) (47.9263, -711.0172) (48.0939, -711.4308) (48.2641, -711.8437) (48.4369, -712.2559) (48.6124, -712.6674) (48.7905, -713.0781) (48.9711, -713.4882) (49.1542, -713.8976) (49.3397, -714.3062) (49.5277, -714.7142) (49.718, -715.1215) (49.9107, -715.5281) (50.1056, -715.934) (50.3027, -716.3392) (50.5021, -716.7438) (50.7037, -717.1476) (50.9074, -717.5508) (51.1132, -717.9534) (51.3211, -718.3552) (51.5311, -718.7564) (51.7432, -719.1569) (51.9573, -719.5567) (52.1734, -719.9559) (52.3914, -720.3544) (52.6114, -720.7522) (52.8333, -721.1494) (53.0572, -721.5459) (53.2829, -721.9417) (53.5106, -722.3369) (53.74, -722.7314) (53.9713, -723.1252) (54.2045, -723.5184) (54.4394, -723.9109) (54.6761, -724.3028) (54.9146, -724.694) (55.1548, -725.0845) (55.3968, -725.4744) (55.6405, -725.8636) (55.8859, -726.2521) (56.1331, -726.64) (56.3819, -727.0273) (56.6323, -727.4138) (56.8845, -727.7997) (57.1382, -728.185) (57.3936, -728.5696) (57.6506, -728.9535) (57.9092, -729.3367) (58.1694, -729.7193) (58.4312, -730.1013) (58.6419, -730.4063) (58.8007, -730.6348) (58.9068, -730.7869) (58.96, -730.863) knots 0.10707295 0.10707295 0.10707295 0.10707295 0.10707295 0.10707295 0.11428571 0.12857143 0.14285714 0.15714286 0.17142857 0.18571429 0.2 0.21428571 0.22857143 0.24285714 0.25714286 0.27142857 0.28571429 0.3 0.31428571 0.32857143 0.34285714 0.35714286 0.37142857 0.38571429 0.4 0.41428571 0.42857143 0.44285714 0.45714286 0.47142857 0.48571429 0.5 0.51428571 0.52857143 0.54285714 0.55714286 0.57142857 0.58571429 0.6 0.61428571 0.62857143 0.64285714 0.65714286 0.67142857 0.68571429 0.7 0.71428571 0.72857143 0.74285714 0.75714286 0.77142857 0.78571429 0.8 0.81428571 0.82857143 0.84285714 0.85714286 0.87142857 0.88571429 0.9 0.91428571 0.92857143 0.94285714 0.95714286 0.97142857 0.98571429 1 1 1 1 1 1
  arc A27 (58.96, -730.863) -> (68.5748, -729.1676) centre (11.949, -436.1388) ccw
  spline S54 degree 5 poles (68.5748, -729.1676) (68.5987, -729.078) (68.6464, -728.8987) (68.7174, -728.6297) (68.8111, -728.271) (68.9265, -727.8226) (69.0401, -727.3741) (69.1521, -726.9255) (69.2623, -726.4768) (69.3707, -726.0281) (69.4774, -725.5793) (69.5824, -725.1304) (69.6855, -724.6815) (69.7869, -724.2325) (69.8864, -723.7835) (69.9841, -723.3344) (70.08, -722.8853) (70.1741, -722.4362) (70.2662, -721.9871) (70.3566, -721.5379) (70.445, -721.0887) (70.5315, -720.6395) (70.6161, -720.1903) (70.6987, -719.7411) (70.7794, -719.2919) (70.8582, -718.8427) (70.9349, -718.3935) (71.0097, -717.9444) (71.0824, -717.4953) (71.153, -717.0462) (71.2216, -716.5971) (71.2882, -716.1481) (71.3526, -715.6992) (71.4149, -715.2503) (71.475, -714.8015) (71.533, -714.3528) (71.5887, -713.9042) (71.6422, -713.4556) (71.6935, -713.0072) (71.7425, -712.5588) (71.7891, -712.1106) (71.8335, -711.6625) (71.8754, -711.2146) (71.915, -710.7667) (71.9521, -710.3191) (71.9867, -709.8716) (72.0188, -709.4243) (72.0482, -708.9772) (72.075, -708.5303) (72.0992, -708.0836) (72.1207, -707.6371) (72.1394, -707.1909) (72.1553, -706.7449) (72.1684, -706.2992) (72.1786, -705.8538) (72.1856, -705.4087) (72.1895, -704.964) (72.19, -704.5196) (72.187, -704.0757) (72.1807, -703.6321) (72.1709, -703.189) (72.1577, -702.7463) (72.141, -702.304) (72.1226, -701.906) (72.1057, -701.5966) (72.0922, -701.3758) (72.0835, -701.2432) (72.0805, -701.1987) knots -1 -1 -1 -1 -1 -1 -0.98571429 -0.97142857 -0.95714286 -0.94285714 -0.92857143 -0.91428571 -0.9 -0.88571429 -0.87142857 -0.85714286 -0.84285714 -0.82857143 -0.81428571 -0.8 -0.78571429 -0.77142857 -0.75714286 -0.74285714 -0.72857143 -0.71428571 -0.7 -0.68571429 -0.67142857 -0.65714286 -0.64285714 -0.62857143 -0.61428571 -0.6 -0.58571429 -0.57142857 -0.55714286 -0.54285714 -0.52857143 -0.51428571 -0.5 -0.48571429 -0.47142857 -0.45714286 -0.44285714 -0.42857143 -0.41428571 -0.4 -0.38571429 -0.37142857 -0.35714286 -0.34285714 -0.32857143 -0.31428571 -0.3 -0.28571429 -0.27142857 -0.25714286 -0.24285714 -0.22857143 -0.21428571 -0.2 -0.18571429 -0.17142857 -0.15714286 -0.14285714 -0.12857143 -0.11428571 -0.10707295 -0.10707295 -0.10707295 -0.10707295 -0.10707295 -0.10707295
  spline S55 degree 3 poles (73.3043, -699.5466) (73.103, -699.5935) (72.9128, -699.6793) (72.5759, -699.9189) (72.4324, -700.0705) (72.2329, -700.3865) (72.1666, -700.5409) (72.0846, -700.8647) (72.0694, -701.0321) (72.0805, -701.1987) knots 0 0 0 0 0.062015 0.062015 0.12403 0.12403 0.174133 0.174133 0.224236 0.224236 0.224236 0.224236
  arc A28 (73.3043, -699.5466) -> (81.438, -697.5187) centre (11.949, -436.1388) ccw
  spline S56 degree 3 poles (83.2942, -698.4028) (83.2095, -698.2143) (83.0888, -698.044) (82.789, -697.7593) (82.6127, -697.6476) (82.2643, -697.5125) (82.1001, -697.477) (81.7665, -697.4586) (81.5994, -697.4758) (81.438, -697.5187) knots 0 0 0 0 0.062015 0.062015 0.12403 0.12403 0.174133 0.174133 0.224236 0.224236 0.224236 0.224236
  spline S57 degree 5 poles (83.2942, -698.4028) (83.3124, -698.4435) (83.367, -698.5647) (83.4587, -698.766) (83.589, -699.0471) (83.7596, -699.4072) (83.9525, -699.8055) (84.1487, -700.2026) (84.3481, -700.5984) (84.5507, -700.993) (84.7566, -701.3864) (84.9656, -701.7785) (85.1778, -702.1694) (85.393, -702.5591) (85.6111, -702.9476) (85.8319, -703.335) (86.0553, -703.7213) (86.2814, -704.1065) (86.5099, -704.4906) (86.7409, -704.8737) (86.9744, -705.2557) (87.2103, -705.6366) (87.4487, -706.0165) (87.6893, -706.3954) (87.9322, -706.7732) (88.1774, -707.15) (88.4247, -707.5258) (88.6742, -707.9007) (88.9259, -708.2745) (89.1796, -708.6474) (89.4354, -709.0193) (89.6932, -709.3902) (89.9531, -709.7602) (90.2149, -710.1291) (90.4787, -710.4972) (90.7444, -710.8643) (91.0121, -711.2304) (91.2816, -711.5956) (91.553, -711.9599) (91.8262, -712.3232) (92.1013, -712.6857) (92.3781, -713.0471) (92.6568, -713.4077) (92.9372, -713.7674) (93.2193, -714.1261) (93.5032, -714.4839) (93.7888, -714.8408) (94.076, -715.1968) (94.365, -715.5519) (94.6556, -715.9061) (94.9478, -716.2594) (95.2417, -716.6118) (95.5372, -716.9633) (95.8343, -717.3139) (96.133, -717.6637) (96.4333, -718.0125) (96.7351, -718.3605) (97.0385, -718.7075) (97.3434, -719.0537) (97.6499, -719.399) (97.9578, -719.7434) (98.2672, -720.0869) (98.5781, -720.4296) (98.8905, -720.7714) (99.1416, -721.0441) (99.3306, -721.2483) (99.4569, -721.3842) (99.5201, -721.4521) knots 0.10707295 0.10707295 0.10707295 0.10707295 0.10707295 0.10707295 0.11428571 0.12857143 0.14285714 0.15714286 0.17142857 0.18571429 0.2 0.21428571 0.22857143 0.24285714 0.25714286 0.27142857 0.28571429 0.3 0.31428571 0.32857143 0.34285714 0.35714286 0.37142857 0.38571429 0.4 0.41428571 0.42857143 0.44285714 0.45714286 0.47142857 0.48571429 0.5 0.51428571 0.52857143 0.54285714 0.55714286 0.57142857 0.58571429 0.6 0.61428571 0.62857143 0.64285714 0.65714286 0.67142857 0.68571429 0.7 0.71428571 0.72857143 0.74285714 0.75714286 0.77142857 0.78571429 0.8 0.81428571 0.82857143 0.84285714 0.85714286 0.87142857 0.88571429 0.9 0.91428571 0.92857143 0.94285714 0.95714286 0.97142857 0.98571429 1 1 1 1 1 1
  arc A29 (99.5201, -721.4521) -> (108.8054, -718.4351) centre (11.949, -436.1388) ccw
  spline S58 degree 5 poles (108.8054, -718.4351) (108.8167, -718.343) (108.8389, -718.1588) (108.8718, -717.8826) (108.9147, -717.5143) (108.9665, -717.0542) (109.0167, -716.5942) (109.0651, -716.1344) (109.1118, -715.6748) (109.1567, -715.2153) (109.1999, -714.756) (109.2413, -714.2969) (109.281, -713.838) (109.3189, -713.3793) (109.355, -712.9208) (109.3893, -712.4625) (109.4217, -712.0045) (109.4523, -711.5466) (109.4811, -711.089) (109.508, -710.6316) (109.5331, -710.1745) (109.5562, -709.7177) (109.5775, -709.261) (109.5968, -708.8047) (109.6142, -708.3486) (109.6297, -707.8929) (109.6431, -707.4374) (109.6546, -706.9822) (109.6641, -706.5273) (109.6716, -706.0728) (109.6771, -705.6186) (109.6805, -705.1647) (109.6818, -704.7112) (109.681, -704.258) (109.6781, -703.8052) (109.673, -703.3528) (109.6658, -702.9007) (109.6564, -702.4491) (109.6447, -701.9979) (109.6308, -701.5471) (109.6146, -701.0967) (109.5962, -700.6468) (109.5754, -700.1974) (109.5522, -699.7484) (109.5267, -699.3) (109.4987, -698.852) (109.4682, -698.4046) (109.4351, -697.9577) (109.3995, -697.5114) (109.3612, -697.0658) (109.3203, -696.6207) (109.2768, -696.1762) (109.2305, -695.7323) (109.1814, -695.2891) (109.1295, -694.8466) (109.0745, -694.4049) (109.0164, -693.9639) (108.9551, -693.5238) (108.8904, -693.0846) (108.8224, -692.6463) (108.751, -692.2088) (108.6764, -691.7722) (108.5983, -691.3366) (108.5246, -690.945) (108.4648, -690.641) (108.4207, -690.4242) (108.3937, -690.2941) (108.3845, -690.2505) knots -1 -1 -1 -1 -1 -1 -0.98571429 -0.97142857 -0.95714286 -0.94285714 -0.92857143 -0.91428571 -0.9 -0.88571429 -0.87142857 -0.85714286 -0.84285714 -0.82857143 -0.81428571 -0.8 -0.78571429 -0.77142857 -0.75714286 -0.74285714 -0.72857143 -0.71428571 -0.7 -0.68571429 -0.67142857 -0.65714286 -0.64285714 -0.62857143 -0.61428571 -0.6 -0.58571429 -0.57142857 -0.55714286 -0.54285714 -0.52857143 -0.51428571 -0.5 -0.48571429 -0.47142857 -0.45714286 -0.44285714 -0.42857143 -0.41428571 -0.4 -0.38571429 -0.37142857 -0.35714286 -0.34285714 -0.32857143 -0.31428571 -0.3 -0.28571429 -0.27142857 -0.25714286 -0.24285714 -0.22857143 -0.21428571 -0.2 -0.18571429 -0.17142857 -0.15714286 -0.14285714 -0.12857143 -0.11428571 -0.10707295 -0.10707295 -0.10707295 -0.10707295 -0.10707295 -0.10707295
  spline S59 degree 3 poles (109.3665, -688.4441) (109.1737, -688.5186) (108.9972, -688.63) (108.697, -688.9142) (108.576, -689.0843) (108.4224, -689.425) (108.3783, -689.5871) (108.3421, -689.9192) (108.3503, -690.087) (108.3845, -690.2505) knots 0 0 0 0 0.062015 0.062015 0.12403 0.12403 0.174133 0.174133 0.224236 0.224236 0.224236 0.224236
  arc A30 (109.3665, -688.4441) -> (117.1388, -685.304) centre (11.949, -436.1388) ccw
  spline S60 degree 3 poles (119.0999, -685.9212) (118.9899, -685.7462) (118.8467, -685.5944) (118.5102, -685.3542) (118.3201, -685.2682) (117.9562, -685.1828) (117.7886, -685.1705) (117.4558, -685.1987) (117.2926, -685.239) (117.1388, -685.304) knots 0 0 0 0 0.062015 0.062015 0.12403 0.12403 0.174133 0.174133 0.224236 0.224236 0.224236 0.224236
  spline S61 degree 5 poles (119.0999, -685.9212) (119.1237, -685.9589) (119.1946, -686.0713) (119.3135, -686.2579) (119.4816, -686.5181) (119.7007, -686.8509) (119.9471, -687.2186) (120.1966, -687.5845) (120.4492, -687.9487) (120.7048, -688.3113) (120.9634, -688.6722) (121.225, -689.0314) (121.4895, -689.3889) (121.7568, -689.7449) (122.0268, -690.0992) (122.2994, -690.4521) (122.5744, -690.8036) (122.8519, -691.1536) (123.1316, -691.5021) (123.4137, -691.8493) (123.6981, -692.1951) (123.9848, -692.5395) (124.2736, -692.8825) (124.5646, -693.2242) (124.8578, -693.5646) (125.153, -693.9036) (125.4503, -694.2414) (125.7495, -694.5778) (126.0507, -694.913) (126.3538, -695.2469) (126.6589, -695.5796) (126.9659, -695.911) (127.2747, -696.2412) (127.5853, -696.5702) (127.8978, -696.8979) (128.212, -697.2245) (128.528, -697.5498) (128.8457, -697.8739) (129.1652, -698.1969) (129.4863, -698.5187) (129.8091, -698.8393) (130.1336, -699.1587) (130.4597, -699.477) (130.7874, -699.7941) (131.1167, -700.1101) (131.4477, -700.4249) (131.7801, -700.7386) (132.1141, -701.0512) (132.4497, -701.3626) (132.7868, -701.6729) (133.1254, -701.9821) (133.4654, -702.2902) (133.807, -702.5971) (134.15, -702.903) (134.4944, -703.2077) (134.8403, -703.5114) (135.1877, -703.8139) (135.5364, -704.1154) (135.8865, -704.4158) (136.238, -704.7151) (136.5909, -705.0133) (136.9451, -705.3104) (137.3007, -705.6065) (137.6576, -705.9014) (137.9443, -706.1366) (138.1598, -706.3124) (138.3038, -706.4294) (138.3758, -706.4879) knots 0.10707295 0.10707295 0.10707295 0.10707295 0.10707295 0.10707295 0.11428571 0.12857143 0.14285714 0.15714286 0.17142857 0.18571429 0.2 0.21428571 0.22857143 0.24285714 0.25714286 0.27142857 0.28571429 0.3 0.31428571 0.32857143 0.34285714 0.35714286 0.37142857 0.38571429 0.4 0.41428571 0.42857143 0.44285714 0.45714286 0.47142857 0.48571429 0.5 0.51428571 0.52857143 0.54285714 0.55714286 0.57142857 0.58571429 0.6 0.61428571 0.62857143 0.64285714 0.65714286 0.67142857 0.68571429 0.7 0.71428571 0.72857143 0.74285714 0.75714286 0.77142857 0.78571429 0.8 0.81428571 0.82857143 0.84285714 0.85714286 0.87142857 0.88571429 0.9 0.91428571 0.92857143 0.94285714 0.95714286 0.97142857 0.98571429 1 1 1 1 1 1
  arc A31 (138.3758, -706.4879) -> (147.1509, -702.208) centre (11.949, -436.1388) ccw